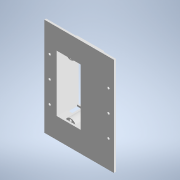
# Autodesk Inventor part: battery_case
Saved by Autodesk Inventor 2022 (Build 260153000, 153)
## iProperties
Created: 2022-10-11
Part Number: battery_case
Material: Типовые
Document SubType Name: Modeling
Designer: korsh624
Density: 1 g/cm^3
Appearance: По умолчанию
Author: korsh624
Autodesk Inventor part; units mm, degrees
ref_plane "YZ Plane" through (0, 0, 0) normal (1, 0, 0) x (0, 1, 0)
ref_plane "XZ Plane" through (0, 0, 0) normal (0, 1, 0) x (-1, 0, 0)
ref_plane "XY Plane" through (0, 0, 0) normal (0, 0, 1) x (1, 0, 0)
sketch "Эскиз1" plane through (0, 0, 0) normal (0, 0, 1) x (1, 0, 0)
  line L0 (126.0318, 90) -> (126.0318, -90) projected
  line L1 (-2.0004, 19) -> (-2.0004, 90) projected
  circle A0 centre (8.0003, 40) radius 2 projected
  circle A1 centre (8.0003, 0) radius 2 projected
  circle A2 centre (8.0003, -40) radius 2 projected
  circle A3 centre (116.0319, 40) radius 2 projected
  circle A4 centre (116.0319, 0) radius 2 projected
  circle A5 centre (116.0319, -40) radius 2 projected
  line L2 (-2, -79) -> (-2, 19) projected
  line L3 (-2.0004, -90) -> (-2.0004, -79) projected
  line L4 (126.0318, 90) -> (-2.0004, 90)
  line L5 (-2.0004, 90) -> (-2.0004, -90)
  line L6 (-2.0004, -90) -> (126.0318, -90)
  line L7 (126.0318, -90) -> (126.0318, 90)
  line L8 (68.0384, 55) -> (18.0384, 55)
  line L9 (18.0384, 55) -> (18.0384, -55)
  line L10 (18.0384, -55) -> (68.0384, -55)
  line L11 (68.0384, -55) -> (68.0384, 55)
  point P0 (0, 0)
  dimension "d0" = 50
  dimension "d1" = 110
  dimension "d2" = 180
  dimension "d3" = 35
  constraints: 16 end point, 4 parallel, 2 horizontal, 2 perpendicular
  measures "d0" distance of L9.end L10.end
  measures "d1" distance of L10.end L8.start
  measures "d2" distance between parallel lines of L6 L4
  measures "d3" distance between parallel lines of L10 L6
extrude "Выдавливание1" add sketch "Эскиз1" along normal blind 3.5
sketch "Эскиз2" plane through (0, 0, 3.5) normal (0, 0, 1) x (1, 0, 0)
  line L0 (18.0384, -55) -> (18.0384, 55) projected
  line L1 (18.0384, 55) -> (68.0384, 55) projected
  line L2 (68.0384, 55) -> (68.0384, -55) projected
  line L3 (68.0384, -55) -> (18.0384, -55) projected
  line L4 (65.0384, 52) -> (21.0384, 52)
  line L5 (21.0384, 52) -> (21.0384, -52)
  line L6 (21.0384, -52) -> (65.0384, -52)
  line L7 (65.0384, -52) -> (65.0384, 52)
  point P0 (0, 0)
  dimension "d6" = 3
  dimension "d7" = 3
  dimension "d8" = 3
  dimension "d9" = 3
  constraints: 8 end point, 2 parallel, 1 horizontal, 1 perpendicular
  measures "d6" distance between parallel lines of L5 L0
  measures "d7" distance between parallel lines of L7 L2
  measures "d8" distance between parallel lines of L6 L3
  measures "d9" distance between parallel lines of L1 L4
extrude "Выдавливание2" add sketch "Эскиз2" against normal blind 40
sketch "Эскиз3" plane through (0, 0, -36.5) normal (0, 0, -1) x (-1, 0, 0)
  line L0 (-65.0384, -52) -> (-21.0384, -52) projected
  arc A0 (-34.3523, -52) -> (-51.7245, -52) centre (-43.0384, -55.6937) ccw
  circle A1 centre (-43.0384, -49.8387) radius 2
  line L1 (0, 0) -> (-84.8604, 0) construction
  arc A2 (-51.7245, 52) -> (-34.3523, 52) centre (-43.0384, 55.6937) ccw
  circle A3 centre (-43.0384, 49.8387) radius 2
  line L2 (-34.3523, -52) -> (-51.7245, -52)
  line L3 (-51.7245, 52) -> (-34.3523, 52)
  line L4 (-21.0384, 52) -> (-65.0384, 52) projected
  dimension "d12" = 44
  dimension "d13" = 22
  dimension "d14" = 4
  constraints: 6 end point, 4 centre point, 4 point on circle, 4 symmetric about line, 2 collinear, 2 point on line, 1 horizontal, 2 other
  measures "d12" distance of L0.start L0.end
  measures "d13" horizontal distance of L0.end A0.centre
  measures "d14" diameter of A1
extrude "Выдавливание3" add sketch "Эскиз3" against normal blind 36.5
sketch "Эскиз4" plane through (21.0384, -52, 3.5) normal (0, 1, 0) x (1, 0, 0)
  line L0 (0, 0) -> (0, 40) projected
  line L1 (0, 37.0435) -> (9.3788, 37.0435)
  line L2 (9.3788, 37.0435) -> (9.3788, 18.9873)
  line L3 (9.3788, 18.9873) -> (0, 18.9873)
  line L4 (0, 18.9873) -> (0, 37.0435)
  point P0 (-21.0384, 3.5)
  constraints: 8 end point, 2 parallel, 1 horizontal, 1 perpendicular, 1 point on line
extrude "Выдавливание4" cut sketch "Эскиз4" against normal blind 4
equation "\"d3\" = -0.5 * d1 + 0.5 * d2"
